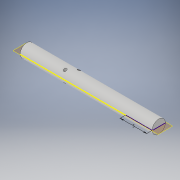
# Autodesk Inventor part: cylindre1
Saved by Autodesk Inventor 2017 (Build 210142000, 142)
## iProperties
Created: 2018-11-09
Part Number: cylindre1
Material: Generic
Document SubType Name: Modeling
Designer: Antoine Blaud
Density: 1 g/cm^3
Appearance: Default
Author: Antoine Blaud
Autodesk Inventor part; units mm, degrees
ref_plane "YZ Plane" through (0, 0, 0) normal (1, 0, 0) x (0, 1, 0)
ref_plane "XY Plane" through (0, 0, 0) normal (0, 0, 1) x (1, 0, 0)
sketch "Sketch1" plane through (0, 0, 0) normal (1, 0, 0) x (0, 1, 0)
  circle A0 centre (0, 0) radius 12.5
  dimension "d0" = 25
  constraints: 1 centre point, 1 coincident
  measures "d0" diameter of A0
extrude "Extrusion1" add sketch "Sketch1" along normal blind 250
sketch "Sketch3" plane through (0, 0, 0) normal (0, 1, 0) x (-1, 0, 0)
  line L0 (-250, 12.5) -> (-250, -12.5) projected
  line L1 (0, -12.5) -> (-250, -12.5) projected
  line L2 (-250, 12.5) -> (-200, 12.5)
  line L3 (-200, 12.5) -> (-200, -12.5)
  line L4 (-200, -12.5) -> (-250, -12.5)
  line L5 (-250, -12.5) -> (-250, 12.5)
  line L6 (-250, 12.5) -> (-200, -12.5)
  line L7 (-200, 12.5) -> (-250, -12.5)
  line L8 (-225, 0) -> (-250, 0)
  line L9 (-225, 0) -> (-200, 0)
  line L10 (0, 12.5) -> (-250, 12.5) projected
  line L11 (-212.5, 12.5) -> (-212.5, -12.5)
  line L12 (-237.5, 12.5) -> (-237.5, -12.5)
  point P0 (0, 0)
  dimension "d5" = 50
  constraints: 20 end point, 5 point on line, 3 midpoint, 3 parallel, 2 perpendicular, 1 horizontal
  measures "d5" distance between parallel lines of L0 L3
sketch "Sketch4" plane through (0, 0, 0) normal (0, 1, 0) x (-1, 0, 0)
  line L0 (0, 12.5) -> (-50, 12.5)
  line L1 (-50, 12.5) -> (-50, -12.5)
  line L2 (-50, -12.5) -> (0, -12.5)
  line L3 (0, -12.5) -> (0, 12.5)
  line L4 (-50, 12.5) -> (0, -12.5)
  line L5 (0, 12.5) -> (-50, -12.5)
  line L6 (-25, 12.5) -> (-25, 0)
  line L7 (-25, 0) -> (-25, -12.5)
  line L8 (0, 0) -> (-50, 0)
  line L9 (-50, 12.5) -> (-108.1359, 12.5)
  line L10 (-108.1359, 12.5) -> (-108.1359, -12.5)
  line L11 (-108.1359, -12.5) -> (-50, -12.5)
  line L12 (-50, -12.5) -> (-50, 12.5)
  line L13 (-108.1359, 12.5) -> (-50, -12.5)
  line L14 (-50, 12.5) -> (-108.1359, -12.5)
  line L15 (-79.068, 12.5) -> (-79.068, -12.5)
  circle A0 centre (-92.5166, -6.25) radius 2.5
  circle A1 centre (-79.068, 6.25) radius 2.5
  circle A2 centre (-79.068, 6.25) radius 8.5
  circle A3 centre (-92.5166, -6.25) radius 8.5
  point P0 (-31.25, 12.5)
  point P1 (-31.25, -12.5)
  point P2 (-50, -6.25)
  point P3 (-50, 6.25)
  point P4 (-37.5, 6.25)
  point P5 (-37.5, -6.25)
  point P6 (-37.5, 6.25)
  point P7 (-64.534, 6.25)
  point P8 (-64.534, -6.25)
  point P9 (-62.5, -12.5)
  point P10 (-62.5, 12.5)
  point P11 (-79.068, -6.25)
  point P12 (-108.1359, -6.25)
  point P13 (-108.1359, 6.25)
  point P14 (-93.6019, 6.25)
  dimension "d6" = 50
  dimension "d7" = 25
  dimension "d8" = 0
  dimension "d9" = 12.5
  dimension "d10" = 108.1359
  dimension "d11" = 25
  dimension "d12" = 31.25
  dimension "d13" = 31.25
  dimension "d14" = 37.5
  dimension "d15" = 37.5
  dimension "d16" = 6.25
  dimension "d17" = 6.25
  dimension "d18" = 5
  dimension "d19" = 5
  dimension "d20" = 17
  dimension "d21" = 17
  dimension "d22" = 62.5
  dimension "d23" = 62.5
  dimension "d24" = 64.534
  dimension "d25" = 64.534
  dimension "d26" = 6.25
  dimension "d27" = 6.25
  dimension "d28" = 92.5166
  dimension "d29" = 6.25
  dimension "d30" = 93.6019
  dimension "d31" = 6.25
  dimension "d32" = 6.25
  constraints: 32 end point, 15 point on line, 7 midpoint, 5 coincident, 4 centre point, 4 parallel, 2 horizontal, 2 perpendicular
  measures "d6" distance between parallel lines of L1 L3
  measures "d7" distance between parallel lines of L0 L2
  measures "d8" distance from line of L8.start L3
  measures "d9" distance from line of L8.start L0
  measures "d10" distance between parallel lines of L10 L3
  measures "d11" distance between parallel lines of L11 L0
  measures "d12" distance from line of point (-31.25, 12.5) L3
  measures "d13" distance from line of point (-31.25, -12.5) L3
  measures "d14" distance from line of point (-37.5, 6.25) L3
  measures "d15" distance from line of point (-37.5, -6.25) L3
  measures "d16" distance from line of point (-50, 6.25) L8
  measures "d17" distance from line of point (-50, -6.25) L8
  measures "d18" diameter of A0
  measures "d19" diameter of A1
  measures "d20" diameter of A2
  measures "d21" diameter of A3
  measures "d22" distance from line of point (-62.5, 12.5) L3
  measures "d23" distance from line of point (-62.5, -12.5) L3
  measures "d24" distance from line of point (-64.534, 6.25) L3
  measures "d25" distance from line of point (-64.534, -6.25) L3
  measures "d26" distance from line of point (-79.068, 6.25) L8
  measures "d27" distance from line of point (-79.068, -6.25) L8
  measures "d28" distance from line of point (-92.517, -6.25) L3
  measures "d29" distance from line of point (-92.517, -6.25) L8
  measures "d30" distance from line of point (-93.602, 6.25) L3
  measures "d31" distance from line of point (-108.136, 6.25) L8
  measures "d32" distance from line of point (-108.136, -6.25) L8
extrude "Extrusion3" cut sketch "Sketch4" along normal mid plane 40 contours A1 L15 | L15 A1 | A0 L14 | L14 A0
body "Solid1"
